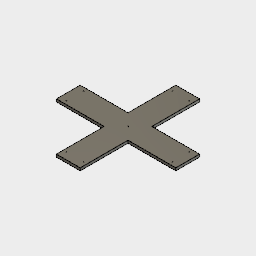
_pendulum_3D.12d040be-d2c6-4b73-b759-7a2067bdbaf2 (Autodesk Fusion 360 design; units mm, degrees)
Autodesk Fusion 360 part; units mm, degrees
sketch "Sketch1" plane through (0, 0, 0) normal (0, 1, 0) x (1, 0, 0)
  line L0 (17.5, -87.5) -> (-17.5, -87.5)
  line L1 (-17.5, 87.5) -> (17.5, 87.5)
  line L2 (17.5, -87.5) -> (-17.5, 87.5) construction
  line L3 (-17.5, -87.5) -> (17.5, 87.5) construction
  line L4 (-87.5, 17.5) -> (-87.5, -17.5)
  line L5 (87.5, -17.5) -> (87.5, 17.5)
  line L6 (87.5, 17.5) -> (-87.5, -17.5) construction
  line L7 (-87.5, 17.5) -> (87.5, -17.5) construction
  circle A0 centre (-77.5, 12.5) radius 0.5
  circle A1 centre (-77.5, -12.5) radius 0.5
  circle A2 centre (-12.5, -77.5) radius 0.5
  circle A3 centre (12.5, -77.5) radius 0.5
  circle A4 centre (77.5, -12.5) radius 0.5
  circle A5 centre (77.5, 12.5) radius 0.5
  circle A6 centre (-12.5, 77.5) radius 0.5
  circle A7 centre (12.5, 77.5) radius 0.5
  line L8 (-17.5, 87.5) -> (-17.5, 17.5)
  line L9 (17.5, 87.5) -> (17.5, 17.5)
  line L10 (-17.5, -87.5) -> (-17.5, -17.5)
  line L11 (17.5, -87.5) -> (17.5, -17.5)
  line L12 (-87.5, 17.5) -> (-17.5, 17.5)
  line L13 (17.5, 17.5) -> (87.5, 17.5)
  line L14 (87.5, -17.5) -> (17.5, -17.5)
  line L15 (-17.5, -17.5) -> (-87.5, -17.5)
  circle A8 centre (0, 0) radius 0.5
  dimension "d1" = 35
  dimension "d2" = 175
  dimension "d3" = 175
  dimension "d4" = 35
  dimension "d7" = 1
  dimension "d8" = 10
  dimension "d10" = 1
  dimension "d12" = 10
  dimension "d13" = 1
  dimension "d14" = 1
  dimension "d15" = 1
  dimension "d16" = 1
  dimension "d17" = 1
  dimension "d18" = 1
  dimension "d20" = 10
  dimension "d21" = 10
  dimension "d24" = 10
  dimension "d25" = 10
  dimension "d28" = 10
  dimension "d29" = 10
  dimension "d31" = 5
  dimension "d32" = 5
  dimension "d33" = 5
  dimension "d34" = 5
  dimension "d35" = 5
  dimension "d36" = 5
  dimension "d37" = 5
  dimension "d38" = 5
  dimension "d39" = 1
  dimension "d40" = 70
  dimension "d41" = 70
  measures "d1" distance of L1.start L1.end
  measures "d2" distance of L0.end L1.start
  measures "d3" distance of L4.end L5.start
  measures "d4" distance of L4.start L4.end
  measures "d7" diameter of A0
  measures "d8" distance of L4 A0.centre
  measures "d10" diameter of A1
  measures "d12" distance of L4 A1.centre
  measures "d13" diameter of A2
  measures "d14" diameter of A3
  measures "d15" diameter of A4
  measures "d16" diameter of A5
  measures "d17" diameter of A6
  measures "d18" diameter of A7
  measures "d20" distance of L1 A6.centre
  measures "d21" distance of L1 A7.centre
  measures "d24" distance of L5 A5.centre
  measures "d25" distance of L5 A4.centre
  measures "d28" distance of L0 A3.centre
  measures "d29" distance of L0 A2.centre
  measures "d31" distance of A1.centre L15
  measures "d32" distance of A0.centre L12
  measures "d33" distance of A6.centre L8
  measures "d34" distance of A7.centre L9
  measures "d35" distance of A5.centre L13
  measures "d36" distance of A4.centre L14
  measures "d37" distance of A3.centre L11
  measures "d38" distance of A2.centre L10
  measures "d39" diameter of A8
  measures "d40" distance of L4 L8
  measures "d41" distance of L1 L12
extrude "Extrude1" add sketch "Sketch1" along normal blind 3.93
